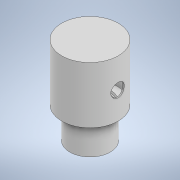
# Autodesk Inventor part: shroud 2
Saved by Autodesk Inventor 2020 (Build 240168000, 168)
## iProperties
Created: 2019-07-24
Part Number: shroud 2
Material: Generic
Document SubType Name: Modeling
Designer: ColinP
Density: 1 g/cm^3
Appearance: Default
Author: ColinP
Autodesk Inventor part; units mm, degrees
ref_plane "YZ Plane" through (0, 0, 0) normal (1, 0, 0) x (0, 1, 0)
ref_plane "XZ Plane" through (0, 0, 0) normal (0, 1, 0) x (-1, 0, 0)
ref_plane "XY Plane" through (0, 0, 0) normal (0, 0, 1) x (1, 0, 0)
sketch "Sketch5" plane through (0, 0, 0) normal (0, 1, 0) x (-1, 0, 0)
  circle A0 centre (0, 0) radius 17.78
  circle A1 centre (0, 0) radius 19.05
  dimension "d16" = 35.56
  dimension "d17" = 38.1
  constraints: 2 centre point, 2 coincident
  measures "d16" diameter of A0
  measures "d17" diameter of A1
extrude "Extrusion5" add sketch "Sketch5" along normal blind 25.4
sketch "Sketch6" plane through (0, 25.4, 0) normal (0, 1, 0) x (1, 0, 0)
  circle A0 centre (0, 0) radius 25.4
  circle A1 centre (0, 0) radius 26.67
  circle A2 centre (0, 0) radius 19.05 projected
  dimension "d20" = 50.8
  dimension "d21" = 53.34
  constraints: 2 centre point, 2 coincident
  measures "d20" diameter of A0
  measures "d21" diameter of A1
extrude "Extrusion6" add sketch "Sketch6" along normal blind 50.8 contours A1
sketch "Sketch7" plane through (0, 76.2, 0) normal (0, 1, 0) x (1, 0, 0)
  circle A0 centre (0, 0) radius 26.67 projected
extrude "Extrusion8" add sketch "Sketch7" along normal blind 2.54
sketch "Sketch8" plane through (0, 0, 0) normal (1, 0, 0) x (0, 1, 0)
  line L0 (0, 0) -> (50.8, 0)
  circle A0 centre (50.8, 0) radius 6.35
  dimension "d28" = 50.8
  dimension "d29" = 12.7
  constraints: 2 end point, 1 centre point, 1 coincident, 1 horizontal
  measures "d28" distance of L0.start L0.end
  measures "d29" diameter of A0
extrude "Extrusion9" cut sketch "Sketch8" along normal mid plane 127
extrude "Extrusion10" add sketch "Sketch6" along normal blind 2.54 contours A0
sketch "Sketch12" plane through (0, 0, 0) normal (0, -1, 0) x (1, 0, 0)
  circle A0 centre (0, 0) radius 19.05 projected
  circle A1 centre (0, 0) radius 17.78 projected
extrude "Extrusion13" add sketch "Sketch12" along normal blind 3.81
body "Solid2"
